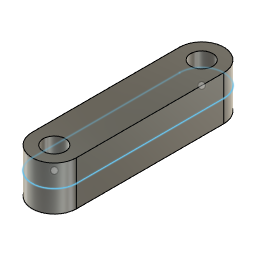
Assembly (Autodesk Fusion 360 archive; units mm, degrees)
design "Link1"
Autodesk Fusion 360 part; units mm, degrees
sketch "Schizzo1" plane through (0, 0, 0) normal (0, 0, 1) x (1, 0, 0)
  line L0 (-150, 150) -> (-150, 1150)
  line L1 (150, 150) -> (150, 1150)
  arc A0 (150, 1150) -> (-150, 1150) centre (0, 1150) ccw
  arc A1 (-150, 150) -> (150, 150) centre (0, 150) ccw
  dimension "d1" = 300
  dimension "d2" = 1000
  dimension "d3" = 1000
  constraint tangent L0 A1
  constraint vertical L0
  constraint tangent L1 A1
  constraint vertical L1
  constraint tangent L1 A0
  measures "d1" diameter of A1
  measures "d2" distance of L0.start L0.end
  measures "d3" distance of L1.start L1.end
extrude "Estrusione1" add sketch "Schizzo1" along normal mid plane 300
sketch "Schizzo2" plane through (0, 0, 150) normal (0, 0, 1) x (-1, 0, 0)
  arc A0 (150, -150) -> (-150, -150) centre (0, -150) ccw
  line L0 (-150, -150) -> (-150, -1150)
  arc A1 (-150, -1150) -> (150, -1150) centre (0, -1150) ccw
  line L1 (150, -1150) -> (150, -150)
  circle A2 centre (0, -150) radius 75
  circle A3 centre (0, -1150) radius 75
  dimension "d6" = 150
  dimension "d7" = 150
  constraint concentric A0 A2
  constraint concentric A1 A3
  measures "d6" diameter of A3
  measures "d7" diameter of A2
extrude "Estrusione2" cut sketch "Schizzo2" against normal blind 300 contours A2 | A3

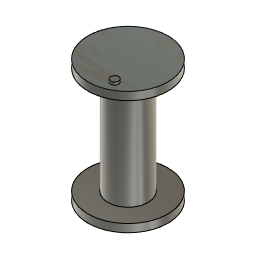
design "Motor"
Autodesk Fusion 360 part; units mm, degrees
sketch "Schizzo1" plane through (0, 0, 0) normal (0, 0, 1) x (1, 0, 0)
  circle A0 centre (0, 0) radius 75
  dimension "d1" = 150
  constraint coincident A0.centre origin
  measures "d1" diameter of A0
extrude "Estrusione1" add sketch "Schizzo1" along normal mid plane 400
sketch "Schizzo2" plane through (0, 0, 200) normal (0, 0, 1) x (-1, 0, 0)
  circle A0 centre (0, 0) radius 75
  circle A1 centre (0, 0) radius 150
  dimension "d4" = 300
  constraint coincident A0.centre A1.centre
  measures "d4" diameter of A1
extrude "Estrusione2" add sketch "Schizzo2" along normal blind 30 contours A0 | A1
sketch "Schizzo3" plane through (0, 0, -200) normal (0, 0, -1) x (1, 0, 0)
  circle A0 centre (0, 0) radius 75
  circle A1 centre (0, 0) radius 150
  circle A2 centre (0, 0) radius 75
  dimension "d7" = 300
  constraint concentric A1 A2
  measures "d7" diameter of A1
extrude "Estrusione3" add sketch "Schizzo3" along normal blind 30 contours A0 A2 | A1
sketch "Schizzo4" plane through (0, 0, 230) normal (0, 0, 1) x (-1, 0, 0)
  circle A0 centre (0, 0) radius 150
sketch "Schizzo5" plane through (0, 0, 230) normal (0, 0, 1) x (-1, 0, 0)
  circle A0 centre (-50, 100) radius 15
  dimension "d10" = 30
  measures "d10" diameter of A0
extrude "Estrusione4" add sketch "Schizzo5" along normal blind 10

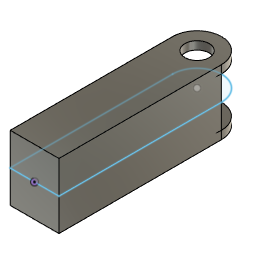
design "Link2"
Autodesk Fusion 360 part; units mm, degrees
sketch "Schizzo1" plane through (0, 0, 0) normal (0, 0, 1) x (1, 0, 0)
  line L0 (-150, 0) -> (-150, 1000)
  line L1 (150, 0) -> (150, 1000)
  arc A0 (150, 1000) -> (-150, 1000) centre (0, 1000) ccw
  line L2 (-150, 0) -> (150, 0)
  dimension "d1" = 150
  dimension "d2" = 150
  dimension "d3" = 1000
  dimension "d4" = 1000
  constraint tangent L1 A0
  constraint perpendicular L1 L2
  measures "d1" distance of origin L0.start
  measures "d2" distance of origin L1.start
  measures "d3" distance of L1.start L1.end
  measures "d4" distance of L0.start L0.end
extrude "Estrusione1" add sketch "Schizzo1" along normal mid plane 400
ref_plane "Piano di lavoro1" through (0, 575, 0) normal (0, 0, 1) x (1, 0, 0)
sketch "Schizzo2" plane through (0, 575, 0) normal (0, 0, 1) x (1, 0, 0)
  circle A0 centre (0, 425) radius 150
  arc A1 (150, 425) -> (-150, 425) centre (0, 425) ccw
  dimension "d7" = 300
  constraint concentric A0 A1
  measures "d7" diameter of A0
extrude "Estrusione2" cut sketch "Schizzo2" along normal mid plane 300
sketch "Schizzo3" plane through (0, 0, 200) normal (0, 0, 1) x (-1, 0, 0)
  line L0 (150, 0) -> (-150, 0)
  line L1 (-150, 0) -> (-150, -1000)
  arc A0 (-150, -1000) -> (150, -1000) centre (0, -1000) ccw
  line L2 (150, -1000) -> (150, 0)
  circle A1 centre (0, -1000) radius 75
  dimension "d10" = 150
  constraint concentric A0 A1
  measures "d10" diameter of A1
extrude "Estrusione3" cut sketch "Schizzo3" against normal blind 400 contours A1

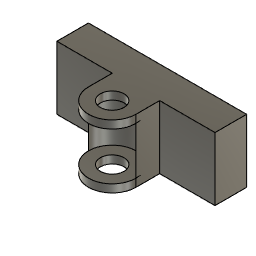
design "Basis"
Autodesk Fusion 360 part; units mm, degrees
sketch "Schizzo1" plane through (0, 0, 0) normal (0, 0, 1) x (1, 0, 0)
  line L0 (-150, 0) -> (-150, 150)
  line L1 (150, 0) -> (150, 150)
  line L2 (150, 150) -> (500, 150)
  line L3 (-150, 150) -> (-500, 150)
  line L4 (-500, 150) -> (-500, 350)
  line L5 (500, 150) -> (500, 350)
  line L6 (500, 350) -> (-500, 350)
  arc A0 (-150, 0) -> (150, 0) centre (0, 0) ccw
  dimension "d1" = 300
  dimension "d2" = 150
  dimension "d3" = 150
  dimension "d4" = 1000
  constraint coincident A0.centre origin
  constraint tangent L0 A0
  constraint vertical L0
  constraint tangent L1 A0
  constraint vertical L1
  constraint perpendicular L1 L2
  constraint perpendicular L0 L3
  constraint perpendicular L3 L4
  constraint perpendicular L2 L5
  constraint perpendicular L5 L6
  measures "d1" diameter of A0
  measures "d2" distance of L1.start L1.end
  measures "d3" distance of L0.start L0.end
  measures "d4" distance of L4.end L5.end
extrude "Estrusione1" add sketch "Schizzo1" along normal mid plane 400
ref_plane "Piano di lavoro1" through (0, 100, 0) normal (0, 0, -1) x (-1, 0, 0)
sketch "Schizzo2" plane through (0, 100, 0) normal (0, 0, -1) x (1, 0, 0)
  circle A0 centre (0, 100) radius 150
  arc A1 (150, 100) -> (-150, 100) centre (0, 100) ccw
  dimension "d7" = 300
  constraint concentric A0 A1
  measures "d7" diameter of A0
extrude "Estrusione2" cut sketch "Schizzo2" along normal mid plane 300
sketch "Schizzo3" plane through (0, 0, 200) normal (0, 0, 1) x (-1, 0, 0)
  line L0 (150, -150) -> (150, 0)
  arc A0 (150, 0) -> (-150, 0) centre (0, 0) ccw
  line L1 (-150, 0) -> (-150, -150)
  line L2 (-150, -150) -> (-500, -150)
  line L3 (-500, -150) -> (-500, -350)
  line L4 (-500, -350) -> (500, -350)
  line L5 (500, -350) -> (500, -150)
  line L6 (500, -150) -> (150, -150)
  circle A1 centre (0, 0) radius 75
  dimension "d10" = 150
  constraint coincident A0.centre A1.centre
  measures "d10" diameter of A1
extrude "Estrusione3" cut sketch "Schizzo3" against normal blind 400 contours A1
